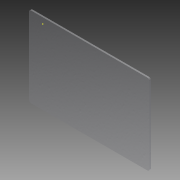
# Autodesk Inventor part: board
Saved by Autodesk Inventor 2015 (Build 190159000, 159)
## iProperties
Created: 2015-01-05
Part Number: board
Material: Acrylic, Clear
Document SubType Name: Modeling
Designer: techlab
Density: 1.19 g/cm^3
Appearance: Transparent - Clear
Author: techlab
Autodesk Inventor part; units mm, degrees
ref_plane "YZ Plane" through (0, 0, 0) normal (1, 0, 0) x (0, 1, 0)
ref_plane "XZ Plane" through (0, 0, 0) normal (0, 1, 0) x (-1, 0, 0)
ref_plane "XY Plane" through (0, 0, 0) normal (0, 0, 1) x (1, 0, 0)
sketch "Sketch1" plane through (0, 0, 0) normal (0, 0, 1) x (1, 0, 0)
  point P0 (0, 0)
sketch "Sketch2" plane through (0, 0, 0) normal (0, 0, 1) x (1, 0, 0)
  line L0 (-15.8604, 11.7809) -> (168.2896, 11.7809)
  line L1 (171.4646, 8.6059) -> (171.4646, -112.0441)
  line L2 (168.2896, -115.2191) -> (-15.8604, -115.2191)
  line L3 (-19.0354, -112.0441) -> (-19.0354, 8.6059)
  arc A0 (-15.8604, 11.7809) -> (-19.0354, 8.6059) centre (-15.8604, 8.6059) ccw
  arc A1 (171.4646, 8.6059) -> (168.2896, 11.7809) centre (168.2896, 8.6059) ccw
  arc A2 (168.2896, -115.2191) -> (171.4646, -112.0441) centre (168.2896, -112.0441) ccw
  arc A3 (-19.0354, -112.0441) -> (-15.8604, -115.2191) centre (-15.8604, -112.0441) ccw
  point P0 (0, 0)
  point P1 (171.4646, -115.2191)
  point P2 (171.4646, 11.7809)
  point P3 (-19.0354, -115.2191)
  dimension "d0" = 190.5
  dimension "d1" = 127
  dimension "d2" = 3.175
  constraints: 8 end point, 8 point on circle, 8 tangent, 6 point on line, 4 centre point, 3 equal radius, 2 parallel, 1 horizontal, 1 perpendicular
  measures "d0" distance of point (171.465, -115.219) point (-19.035, -115.219)
  measures "d1" distance of point (171.465, 11.781) point (171.465, -115.219)
  measures "d2" radius of A0
extrude "Extrusion1" add sketch "Sketch2" along normal blind 2.54
body "Solid1"
